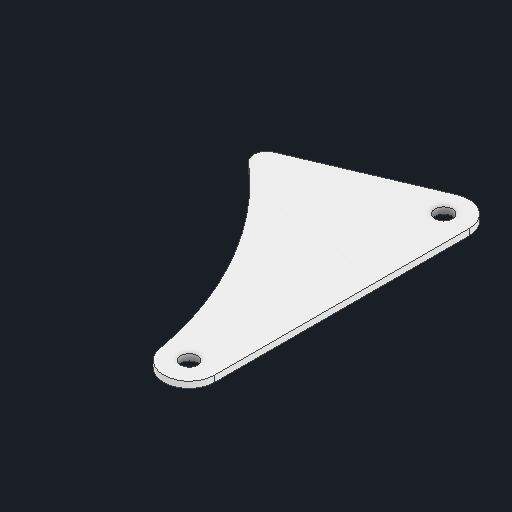
# Autodesk Inventor part: Magazine Gusset
Saved by Autodesk Inventor 2025 (Build 290162000, 162)
## iProperties
Created: 2024-12-31
Part Number: Magazine Gusset
Material: Acetal Resin, White
Document SubType Name: Modeling
Designer: Averey Ku
Density: 1.425 g/cm^3
Appearance: Smooth - White
Author: Averey Ku
Autodesk Inventor part; units mm, degrees
ref_plane "YZ Plane" through (0, 0, 0) normal (1, 0, 0) x (0, 1, 0)
ref_plane "XZ Plane" through (0, 0, 0) normal (0, 1, 0) x (-1, 0, 0)
ref_plane "XY Plane" through (0, 0, 0) normal (0, 0, 1) x (1, 0, 0)
sketch "main" plane through (0, 0, 0) normal (0, 0, 1) x (1, 0, 0)
  circle A0 centre (31.4944, -42.9627) radius 2.1844
  arc A1 (31.4944, -49.3127) -> (37.3322, -40.4642) centre (31.4944, -42.9627) ccw
  arc A2 (-33.1353, -36.714) -> (-32.0056, -49.3127) centre (-32.0056, -42.9627) ccw
  arc A3 (-33.1353, -36.714) -> (18.2379, -7.4459) centre (-48.9511, 50.7679) ccw
  line L0 (37.3322, -40.4642) -> (23.5564, -8.2758)
  line L1 (-32.0056, -49.3127) -> (31.4944, -49.3127)
  arc A4 (23.5564, -8.2758) -> (18.2379, -7.4459) centre (20.6375, -9.525) ccw
  circle A5 centre (-32.0056, -42.9627) radius 2.0955
  point P0 (5.1717, -33.3366)
  point P1 (21.495, -3.459)
  dimension "d0" = 177.8
  dimension "d1" = 12.7
  dimension "d2" = 12.7
  dimension "d3" = 3.175
  dimension "d4" = 4.191
  measures "d0" diameter of A3
  measures "d1" diameter of A2
  measures "d2" diameter of A1
  measures "d3" radius of A4
  measures "d4" diameter of A5
sketch "Sketch1" plane through (0, 0, 0) normal (0, 1, 0) x (-1, 0, 0)
  circle A0 centre (-0.1035, -63.4999) radius 2.1844
  arc A1 (-6.4535, -63.4896) -> (2.3855, -69.3418) centre (-0.1035, -63.4999) ccw
  arc A2 (6.2505, 1.1195) -> (-6.35, 0.0103) centre (0, 0) ccw
  arc A3 (6.2505, 1.1195) -> (35.4348, -50.3013) centre (93.758, 16.7928) ccw
  line L0 (2.3855, -69.3418) -> (34.5963, -55.6185)
  line L1 (-6.35, 0.0103) -> (-6.4535, -63.4896)
  arc A4 (34.5963, -55.6185) -> (35.4348, -50.3013) centre (33.3518, -52.6975) ccw
  circle A5 centre (0, 0) radius 2.0955
  point P0 (0, 0)
  constraints: 1 other
extrude "Extrusion1" add sketch "Sketch1" along normal blind 1.5875
body "Solid1"
